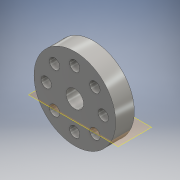
# Autodesk Inventor part: Main Motor to Sprocket Adapter
Saved by Autodesk Inventor 2016 (Build 200138000, 138)
## iProperties
Created: 2016-05-06
Part Number: Main Motor to Sprocket Adapter
Material: Generic
Document SubType Name: Modeling
Designer: Kenneth Daniel
Density: 1 g/cm^3
Appearance: Default
Author: Kenneth Daniel
Autodesk Inventor part; units mm, degrees
ref_plane "YZ Plane" through (0, 0, 0) normal (1, 0, 0) x (0, 1, 0)
ref_plane "XZ Plane" through (0, 0, 0) normal (0, 1, 0) x (-1, 0, 0)
sketch "Sketch1" plane through (0, 0, 0) normal (0, 1, 0) x (-1, 0, 0)
  circle A0 centre (0, 0) radius 14
  line L0 (0, 0) -> (9.779, 0) construction
  circle A1 centre (9.779, 0) radius 1.778
  circle A2 centre (6.9148, 6.9148) radius 1.778
  circle A3 centre (0, 9.779) radius 1.778
  circle A4 centre (-6.9148, 6.9148) radius 1.778
  circle A5 centre (-9.779, 0) radius 1.778
  circle A6 centre (-6.9148, -6.9148) radius 1.778
  circle A7 centre (0, -9.779) radius 1.778
  circle A8 centre (6.9148, -6.9148) radius 1.778
  dimension "d0" = 28
  dimension "d1" = 9.779
  dimension "d2" = 3.556
  dimension "d5" = 360
  constraints: 9 centre point, 2 coincident, 2 end point, 1 horizontal, 17 other
  measures "d0" diameter of A0
  measures "d1" distance of L0.start L0.end
  measures "d2" diameter of A1
extrude "Extrusion1" add sketch "Sketch1" along normal blind 6.4
sketch "Sketch2" plane through (0, 6.4, 0) normal (0, 1, 0) x (1, 0, 0)
  circle A0 centre (0, 0) radius 6.25
  circle A1 centre (0, 0) radius 3
  dimension "d9" = 12.5
  dimension "d10" = 6
  constraints: 2 centre point, 2 coincident
  measures "d9" diameter of A0
  measures "d10" diameter of A1
extrude "Extrusion2" add sketch "Sketch2" along normal blind 4
ref_plane "Work Plane1" through (0, 6.4, -6.25) normal (0, 0, 1) x (1, 0, 0)
sketch "Sketch3" plane through (0, 6.4, -6.25) normal (0, 0, 1) x (1, 0, 0)
  line L0 (-3, 4) -> (3, 4) construction
  line L1 (0, 4) -> (0, 0) construction
  line L2 (-1.778, 0) -> (1.778, 0) construction
  circle A0 centre (0, 2) radius 1.375
  point P0 (0, -6.4)
  dimension "d13" = 2.75
  constraints: 3 midpoint, 2 end point, 1 centre point
  measures "d13" diameter of A0
extrude "Extrusion3" cut sketch "Sketch3" along normal blind 1
sketch "Sketch4" plane through (0, 6.4, 0) normal (0, 1, 0) x (1, 0, 0)
  circle A0 centre (0, 0) radius 3 projected
extrude "Extrusion4" cut sketch "Sketch4" against normal through all
body "Solid1"
